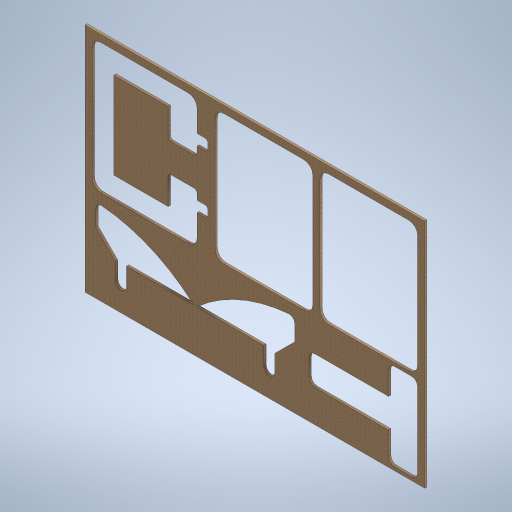
# Autodesk Inventor part: MarcoRompecabezas
Saved by Autodesk Inventor 2023.1 (Build 271208000, 208)
## iProperties
Created: 2022-11-14
Part Number: MarcoRompecabezas
Material: MDF Medium Density Fiberboard
Document SubType Name: Modeling
Designer: Daniel Peña
Density: 0.8 g/cm^3
Appearance: Cardboard - Corrugated
Author: Daniel Peña
Autodesk Inventor part; units mm, degrees
ref_plane "YZ Plane" through (0, 0, 0) normal (1, 0, 0) x (0, 1, 0)
ref_plane "XZ Plane" through (0, 0, 0) normal (0, 1, 0) x (-1, 0, 0)
ref_plane "XY Plane" through (0, 0, 0) normal (0, 0, 1) x (1, 0, 0)
sketch "Sketch1" plane through (0, 0, 0) normal (0, 0, 1) x (1, 0, 0)
  line L0 (24.1957, 7.8063) -> (24.1957, 327.8063)
  line L1 (24.1957, 327.8063) -> (494.1957, 327.8063)
  line L2 (494.1957, 327.8063) -> (494.1957, 7.8063)
  line L3 (494.1957, 7.8063) -> (24.1957, 7.8063)
  arc A0 (70.6957, 42.8063) -> (77.6957, 42.8063) centre (74.1957, 42.8063) ccw
  line L4 (66.6957, 65.6673) -> (66.6957, 42.8063)
  line L5 (39.1957, 93.1673) -> (66.6957, 65.6673)
  line L6 (39.1957, 115.3063) -> (39.1957, 93.1673)
  arc A1 (46.6957, 122.8063) -> (39.1957, 115.3063) centre (46.6957, 115.3063) ccw
  arc A2 (174.1957, 67.8063) -> (46.6957, 122.8063) centre (28.9415, -93.6352) ccw
  line L7 (81.6957, 67.8063) -> (174.1957, 67.8063)
  line L8 (81.6957, 42.8063) -> (81.6957, 67.8063)
  arc A3 (66.6957, 42.8063) -> (81.6957, 42.8063) centre (74.1957, 42.8063) ccw
  circle A4 centre (299.1957, 107.8063) radius 3.5
  line L9 (275.6957, 67.8063) -> (275.6957, 42.8063)
  arc A5 (282.6957, 67.8063) -> (275.6957, 67.8063) centre (279.1957, 67.8063) ccw
  line L10 (282.6957, 42.8063) -> (282.6957, 67.8063)
  arc A6 (275.6957, 42.8063) -> (282.6957, 42.8063) centre (279.1957, 42.8063) ccw
  line L11 (286.6957, 65.6673) -> (286.6957, 42.8063)
  line L12 (314.1957, 93.1673) -> (286.6957, 65.6673)
  line L13 (314.1957, 115.3063) -> (314.1957, 93.1673)
  arc A7 (314.1957, 115.3063) -> (306.6957, 122.8063) centre (306.6957, 115.3063) ccw
  arc A8 (306.6957, 122.8063) -> (179.1957, 67.8063) centre (324.4499, -93.6352) ccw
  line L14 (271.6957, 67.8063) -> (179.1957, 67.8063)
  line L15 (271.6957, 42.8063) -> (271.6957, 67.8063)
  arc A9 (271.6957, 42.8063) -> (286.6957, 42.8063) centre (279.1957, 42.8063) ccw
  circle A10 centre (324.1957, 152.8063) radius 3.5
  circle A11 centre (219.1957, 302.8063) radius 3.5
  circle A12 centre (324.1957, 302.8063) radius 3.5
  circle A13 centre (219.1957, 152.8063) radius 3.5
  line L16 (234.1957, 177.8063) -> (234.1957, 277.8063)
  line L17 (309.1957, 177.8063) -> (234.1957, 177.8063)
  line L18 (309.1957, 277.8063) -> (309.1957, 177.8063)
  line L19 (234.1957, 277.8063) -> (309.1957, 277.8063)
  arc A14 (204.1957, 149.8063) -> (216.1957, 137.8063) centre (216.1957, 149.8063) ccw
  line L20 (204.1957, 305.8063) -> (204.1957, 149.8063)
  arc A15 (216.1957, 317.8063) -> (204.1957, 305.8063) centre (216.1957, 305.8063) ccw
  line L21 (327.1957, 317.8063) -> (216.1957, 317.8063)
  arc A16 (339.1957, 305.8063) -> (327.1957, 317.8063) centre (327.1957, 305.8063) ccw
  line L22 (339.1957, 149.8063) -> (339.1957, 305.8063)
  arc A17 (327.1957, 137.8063) -> (339.1957, 149.8063) centre (327.1957, 149.8063) ccw
  line L23 (216.1957, 137.8063) -> (327.1957, 137.8063)
  circle A18 centre (469.1957, 152.8063) radius 3.5
  circle A19 centre (364.1957, 302.8063) radius 3.5
  circle A20 centre (469.1957, 302.8063) radius 3.5
  circle A21 centre (364.1957, 152.8063) radius 3.5
  line L24 (379.1957, 177.8063) -> (379.1957, 277.8063)
  line L25 (454.1957, 177.8063) -> (379.1957, 177.8063)
  line L26 (454.1957, 277.8063) -> (454.1957, 177.8063)
  line L27 (379.1957, 277.8063) -> (454.1957, 277.8063)
  arc A22 (349.1957, 149.8063) -> (361.1957, 137.8063) centre (361.1957, 149.8063) ccw
  line L28 (349.1957, 305.8063) -> (349.1957, 149.8063)
  arc A23 (361.1957, 317.8063) -> (349.1957, 305.8063) centre (361.1957, 305.8063) ccw
  line L29 (472.1957, 317.8063) -> (361.1957, 317.8063)
  arc A24 (484.1957, 305.8063) -> (472.1957, 317.8063) centre (472.1957, 305.8063) ccw
  line L30 (484.1957, 149.8063) -> (484.1957, 305.8063)
  arc A25 (472.1957, 137.8063) -> (484.1957, 149.8063) centre (472.1957, 149.8063) ccw
  line L31 (361.1957, 137.8063) -> (472.1957, 137.8063)
  circle A26 centre (154.1957, 152.8063) radius 3.5
  circle A27 centre (49.1957, 302.8063) radius 3.5
  circle A28 centre (49.1957, 152.8063) radius 3.5
  circle A29 centre (154.1957, 302.8063) radius 3.5
  circle A30 centre (186.6957, 267.8063) radius 3.5
  circle A31 centre (186.6957, 187.8063) radius 3.5
  arc A32 (139.1957, 251.8063) -> (143.1957, 247.8063) centre (143.1957, 251.8063) ccw
  line L32 (139.1957, 287.8063) -> (139.1957, 251.8063)
  line L33 (64.1957, 287.8063) -> (139.1957, 287.8063)
  line L34 (64.1957, 167.8063) -> (64.1957, 287.8063)
  line L35 (139.1957, 167.8063) -> (64.1957, 167.8063)
  line L36 (139.1957, 203.8063) -> (139.1957, 167.8063)
  arc A33 (143.1957, 207.8063) -> (139.1957, 203.8063) centre (143.1957, 203.8063) ccw
  line L37 (175.1957, 207.8063) -> (143.1957, 207.8063)
  arc A34 (179.1957, 203.8063) -> (175.1957, 207.8063) centre (175.1957, 203.8063) ccw
  line L38 (179.1957, 195.3063) -> (179.1957, 203.8063)
  line L39 (190.1957, 195.3063) -> (179.1957, 195.3063)
  arc A35 (194.1957, 191.3063) -> (190.1957, 195.3063) centre (190.1957, 191.3063) ccw
  line L40 (194.1957, 184.3063) -> (194.1957, 191.3063)
  arc A36 (190.1957, 180.3063) -> (194.1957, 184.3063) centre (190.1957, 184.3063) ccw
  line L41 (179.1957, 180.3063) -> (190.1957, 180.3063)
  line L42 (179.1957, 149.8063) -> (179.1957, 180.3063)
  arc A37 (167.1957, 137.8063) -> (179.1957, 149.8063) centre (167.1957, 149.8063) ccw
  line L43 (46.1957, 137.8063) -> (167.1957, 137.8063)
  arc A38 (34.1957, 149.8063) -> (46.1957, 137.8063) centre (46.1957, 149.8063) ccw
  line L44 (34.1957, 305.8063) -> (34.1957, 149.8063)
  arc A39 (46.1957, 317.8063) -> (34.1957, 305.8063) centre (46.1957, 305.8063) ccw
  line L45 (167.1957, 317.8063) -> (46.1957, 317.8063)
  circle A40 centre (54.1957, 107.8063) radius 3.5
  line L46 (179.1957, 275.3063) -> (179.1957, 305.8063)
  line L47 (190.1957, 275.3063) -> (179.1957, 275.3063)
  arc A41 (194.1957, 271.3063) -> (190.1957, 275.3063) centre (190.1957, 271.3063) ccw
  line L48 (194.1957, 264.3063) -> (194.1957, 271.3063)
  arc A42 (190.1957, 260.3063) -> (194.1957, 264.3063) centre (190.1957, 264.3063) ccw
  line L49 (179.1957, 260.3063) -> (190.1957, 260.3063)
  line L50 (179.1957, 251.8063) -> (179.1957, 260.3063)
  arc A43 (175.1957, 247.8063) -> (179.1957, 251.8063) centre (175.1957, 251.8063) ccw
  line L51 (143.1957, 247.8063) -> (175.1957, 247.8063)
  circle A44 centre (341.6957, 72.8063) radius 3.5
  arc A45 (484.1957, 124.8063) -> (476.1957, 132.8063) centre (476.1957, 124.8063) ccw
  line L52 (484.1957, 20.8063) -> (484.1957, 124.8063)
  arc A46 (476.1957, 12.8063) -> (484.1957, 20.8063) centre (476.1957, 20.8063) ccw
  arc A47 (179.1957, 305.8063) -> (167.1957, 317.8063) centre (167.1957, 305.8063) ccw
  arc A48 (444.1957, 20.8063) -> (452.1957, 12.8063) centre (452.1957, 20.8063) ccw
  line L53 (444.1957, 52.8063) -> (444.1957, 20.8063)
  line L54 (342.1957, 52.8063) -> (444.1957, 52.8063)
  arc A49 (334.1957, 60.8063) -> (342.1957, 52.8063) centre (342.1957, 60.8063) ccw
  line L55 (334.1957, 84.8063) -> (334.1957, 60.8063)
  arc A50 (342.1957, 92.8063) -> (334.1957, 84.8063) centre (342.1957, 84.8063) ccw
  line L56 (444.1957, 92.8063) -> (342.1957, 92.8063)
  line L57 (444.1957, 124.8063) -> (444.1957, 92.8063)
  arc A51 (452.1957, 132.8063) -> (444.1957, 124.8063) centre (452.1957, 124.8063) ccw
  line L58 (476.1957, 132.8063) -> (452.1957, 132.8063)
  line L59 (77.6957, 67.8063) -> (77.6957, 42.8063)
  arc A52 (77.6957, 67.8063) -> (70.6957, 67.8063) centre (74.1957, 67.8063) ccw
  line L60 (70.6957, 42.8063) -> (70.6957, 67.8063)
  line L61 (452.1957, 12.8063) -> (476.1957, 12.8063)
  line L62 (24.1957, 317.8063) -> (494.1957, 317.8063) construction
  line L63 (34.1957, 327.8063) -> (34.1957, 7.8063) construction
  line L64 (24.1957, 17.8063) -> (494.1957, 17.8063) construction
  line L65 (484.1957, 7.8063) -> (484.1957, 327.8063) construction
  point P0 (179.1957, 165.0563)
  point P1 (34.1957, 305.8063)
  point P2 (24.1957, 327.8063)
  point P3 (452.1957, 132.8063)
  point P4 (484.1957, 124.8063)
  point P5 (342.1957, 92.8063)
  point P6 (349.1957, 149.8063)
  point P7 (349.1957, 305.8063)
  point P8 (361.1957, 137.8063)
  point P9 (216.1957, 137.8063)
  point P10 (204.1957, 149.8063)
  point P11 (46.1957, 317.8063)
  dimension "d20" = 30
  dimension "d21" = 30
  dimension "d22" = 30
  dimension "d23" = 40
  dimension "d24" = 4
  dimension "d25" = 4
  dimension "d26" = 4
  dimension "d27" = 4
  dimension "d28" = 7
  dimension "d29" = 7
  dimension "d30" = 7
  dimension "d31" = 7
  dimension "d32" = 75
  dimension "d33" = 12
  dimension "d34" = 12
  dimension "d35" = 12
  dimension "d36" = 12
  dimension "d37" = 120
  dimension "d38" = 40
  dimension "d39" = 25
  dimension "d40" = 15
  dimension "d41" = 15
  dimension "d42" = 15
  dimension "d43" = 15
  dimension "d44" = 15
  dimension "d45" = 10
  dimension "d46" = 10
  dimension "d47" = 10
  dimension "d48" = 10
  dimension "d49" = 140
  dimension "d50" = 5
  dimension "d51" = 50
  dimension "d52" = 145
  dimension "d53" = 12
  dimension "d54" = 123
  dimension "d55" = 145
  dimension "d56" = 22
  dimension "d57" = 12
  dimension "d58" = 13
  constraints: 132 end point, 72 point on circle, 53 centre point, 27 vertical, 24 horizontal, 11 point on line, 4 collinear, 4 perpendicular, 1 midpoint
  measures "d20" distance between parallel lines of L45 L33
  measures "d21" distance between parallel lines of L43 L35
  measures "d22" distance between parallel lines of L34 L44
  measures "d23" distance from line of point (179.196, 165.056) L36
  measures "d24" radius of A32
  measures "d25" radius of A43
  measures "d26" radius of A42
  measures "d27" radius of A41
  measures "d28" diameter of A30
  measures "d29" diameter of A29
  measures "d30" diameter of A27
  measures "d31" diameter of A28
  measures "d32" distance of L35.start L35.end
  measures "d33" radius of A39
  measures "d34" radius of A38
  measures "d35" radius of A37
  measures "d36" radius of A47
  measures "d37" distance between parallel lines of L35 L33
  measures "d38" distance between parallel lines of L51 L37
  measures "d39" distance from line of L46 A29.centre
  measures "d40" distance from line of A29.centre L45
  measures "d41" distance from line of L44 A27.centre
  measures "d42" distance from line of L45 A27.centre
  measures "d43" distance from line of L43 A28.centre
  measures "d44" distance from line of A28.centre L44
  measures "d45" distance between parallel lines of L2 L65
  measures "d46" distance between parallel lines of L1 L62
  measures "d47" distance between parallel lines of L0 L63
  measures "d48" distance between parallel lines of L3 L64
  measures "d49" distance from line of L63 point (174.196, 67.806)
  measures "d50" distance of point (174.196, 67.806) point (179.196, 67.806)
  measures "d51" distance from line of L64 point (174.196, 67.806)
  measures "d52" distance from line of point (179.196, 67.806) L63
  measures "d53" distance from line of L62 point (484.196, 305.806)
  measures "d54" distance from line of L65 A23.start
  measures "d55" distance from line of L65 point (339.196, 305.806)
  measures "d56" distance from line of L1 point (339.196, 305.806)
  measures "d57" distance from line of L62 point (34.196, 305.806)
  measures "d58" distance from line of L3 point (484.196, 20.806)
extrude "Extrusion2" add sketch "Sketch1" along normal blind 3 contours L0 L1 L2 L3
body "Solid2"
